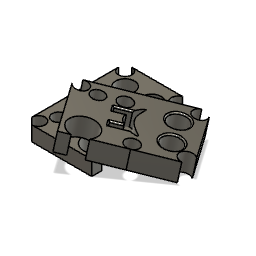
Shape 2 (Autodesk Fusion 360 design; units mm, degrees)
Autodesk Fusion 360 part; units mm, degrees
sketch "Sketch1" plane through (0, 0, 0) normal (0, 1, 0) x (1, 0, 0)
  line L0 (-25, 50) -> (25, 50)
  line L1 (25, 50) -> (25, -25)
  line L2 (25, -25) -> (-25, -25)
  line L3 (-25, -25) -> (-25, 50)
  circle A0 centre (-10, 35) radius 7.0711
  circle A1 centre (10, 35) radius 7.0711
  circle A2 centre (-10, 35) radius 2.5
  circle A3 centre (10, 35) radius 2.5
  spline S0 degree 5 poles (-10, 15) (-9.6, 14.2415) (-8.8, 12.7908) (-7.6, 10.8134) (-6, 8.581) (-4, 6.5094) (-2, 5.2211) (0, 4.7801) (2, 5.2211) (4, 6.5094) (6, 8.581) (7.6, 10.8134) (8.8, 12.7908) (9.6, 14.2415) (10, 15) knots 0 0 0 0 0 0 0.1 0.2 0.3 0.4 0.5 0.6 0.7 0.8 0.9 1 1 1 1 1 1
  line L4 (-8.5952, 12.5) -> (-5, 12.5)
  line L5 (-5, 12.5) -> (-5, 0)
  line L6 (-5, 0) -> (-8.5952, 0)
  line L7 (-8.5952, 0) -> (-8.5952, 12.5)
  line L8 (8.5952, 12.5) -> (5, 12.5)
  line L9 (5, 12.5) -> (5, 0)
  line L10 (5, 0) -> (8.5952, 0)
  line L11 (8.5952, 0) -> (8.5952, 12.5)
  circle A4 centre (-20, -20) radius 5
  circle A5 centre (16.4349, -12.3958) radius 9.9615
  circle A6 centre (-15, -10) radius 4.78
  circle A7 centre (-15, 5) radius 5
  circle A8 centre (20, 45) radius 5.3715
  circle A9 centre (20, 15) radius 5
  circle A10 centre (-20, 45) radius 5
  point P0 (0, 5)
  dimension "d1" = 5
  dimension "d2" = 5
  constraint horizontal L0
  constraint vertical L1
  constraint horizontal L2
  constraint vertical L3
  constraint concentric A0 A2
  constraint concentric A1 A3
  constraint horizontal L4
  constraint vertical L5
  constraint horizontal L6
  constraint vertical L7
  constraint coincident S0 L4.start
  constraint horizontal L8
  constraint vertical L9
  constraint horizontal L10
  constraint vertical L11
  constraint coincident S0 L8.start
  measures "d1" diameter of A2
  measures "d2" diameter of A3
extrude "Extrude1" add sketch "Sketch1" along normal blind 25 contours L0 L1 L2 L3 A4 A5 A8 A10 makes body 1
sketch "Sketch2" plane through (0, 25, 0) normal (0, 1, 0) x (-1, 0, 0)
  circle A0 centre (15, 10) radius 4.78
  circle A1 centre (15, -5) radius 5
  circle A2 centre (10, -35) radius 7.0711
  line L0 (-8.5952, -12.5) -> (-8.5952, 0)
  line L1 (-8.5952, 0) -> (-5, 0)
  line L2 (-5, 0) -> (-5, -12.5)
  line L3 (-5, -12.5) -> (-8.5952, -12.5)
  circle A3 centre (-10, -35) radius 7.0711
  line L4 (5, 0) -> (8.5952, 0)
  line L5 (8.5952, 0) -> (8.5952, -12.5)
  line L6 (8.5952, -12.5) -> (5, -12.5)
  line L7 (5, -12.5) -> (5, 0)
  circle A4 centre (-20, -15) radius 5
  line L8 (-25, -15) -> (-25, -43.0372)
  arc A5 (-18.0372, -50) -> (-25, -43.0372) centre (-20, -45) ccw
  line L9 (-18.0372, -50) -> (20, -50)
  arc A6 (25, -45) -> (20, -50) centre (20, -45) ccw
  line L10 (25, -45) -> (25, 20)
  arc A7 (20, 25) -> (25, 20) centre (20, 20) ccw
  line L11 (20, 25) -> (-25, 25)
  line L12 (-25, 25) -> (-25, 17.4822)
  arc A8 (-25, 7.3095) -> (-25, 17.4822) centre (-16.4349, 12.3958) ccw
  line L13 (-25, 7.3095) -> (-25, -15)
  spline S0 degree 5 poles (12.77, -16.7002) (12.8187, -16.575) (12.7962, -16.1799) (12.4007, -15.1505) (11.1695, -13.0356) (8.6139, -9.9148) (5.282, -7.2489) (1.477, -5.8728) (-2.4553, -6.2838) (-6.1445, -8.3146) (-9.2264, -11.2879) (-11.378, -14.3038) (-12.3547, -16.4917) (-12.0236, -17.244) (-10.4132, -16.538) (-7.7132, -14.9366) (-4.22, -13.2461) (-0.298, -12.2557) (3.6609, -12.4801) (7.2796, -13.8099) (10.2232, -15.5778) (11.8192, -16.6572) (12.5038, -16.9309) (12.7213, -16.8253) (12.77, -16.7002) knots 0 0 0 0 0 0 0.05 0.1 0.15 0.2 0.25 0.3 0.35 0.4 0.45 0.5 0.55 0.6 0.65 0.7 0.75 0.8 0.85 0.9 0.95 1 1 1 1 1 1
  point P0 (0.5135, -6.25)
  point P1 (-12.0217, -16.7002)
  point P2 (1.3491, -12.5)
extrude "Extrude2" cut sketch "Sketch2" against normal blind 45 contours L0 L2 L3 L5 L6 L7 S0 bodies 1
fillet "Fillet1" radius 1 2 edges at (-16.5925, 25, -37.557) (3.4075, 25, -37.557) on bodies 1
fillet "Fillet2" radius 1 2 edges at (-6.7976, 25, 0) (6.7976, 25, 0) on bodies 1
fillet "Fillet3" radius 1 4 edges at (-8.5952, 25, -4.5993) (-5, 25, -3.2395) (5, 25, -3.4428) (8.5952, 25, -4.9308) on bodies 1
sketch "Sketch3" plane through (0, 0, 0) normal (0, 1, 0) x (1, 0, 0)
  line L0 (-40, 60) -> (40, 60)
  line L1 (40, 60) -> (40, -30)
  line L2 (40, -30) -> (-40, -30)
  line L3 (-40, -30) -> (-40, 60)
  constraint horizontal L0
  constraint vertical L1
  constraint horizontal L2
  constraint vertical L3
extrude "Extrude3" add sketch "Sketch3" along normal blind 1 separate body makes body 2
move_body "Move1" bodies 2 to x (1, 0, 0) y (0, 1, 0) z (0, 0, 1) at (0, 10, 0)
split "Split1" by plane through (0, 11, 0) normal (0, 1, 0) bodies 1 makes body 3 at (-2.4997, 25, 7.0631)
move_body "Move2" bodies 3 to x (0.573576, 0, 0.819152) y (0.142244, 0.984808, -0.099601) z (-0.806707, 0.173648, 0.564863) at (12.4443, -1.4342, 3.8466)
hidden bodies 2
